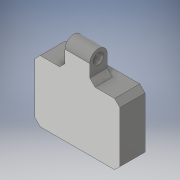
# Autodesk Inventor part: SDCardCover
Saved by Autodesk Inventor 2018 (Build 220112000, 112)
## iProperties
Created: 2019-01-13
Part Number: SDCardCover
Material: Generic
Document SubType Name: Modeling
Designer: tbrow
Density: 1 g/cm^3
Appearance: Default
Author: tbrow
## iProperties of the stored document SDCardCover_3DPrint.ipt
Created: 2019-01-15
Part Number: SDCardCover_3DPrint
Material: Generic
Document SubType Name: Modeling
Designer: tbrow
Density: 1 g/cm^3
Appearance: Default
Author: tbrow
Autodesk Inventor part; units mm, degrees
ref_plane "YZ Plane" through (0, 0, 0) normal (1, 0, 0) x (0, 1, 0)
ref_plane "XZ Plane" through (0, 0, 0) normal (0, 1, 0) x (-1, 0, 0)
ref_plane "XY Plane" through (0, 0, 0) normal (0, 0, 1) x (1, 0, 0)
sketch "Sketch1" plane through (0, 0, 0) normal (0, 0, 1) x (1, 0, 0)
  line L0 (0, 0) -> (0, 22.1234)
  line L1 (0, 22.1234) -> (10.795, 22.1234)
  line L2 (10.795, 22.1234) -> (10.795, 31.6484)
  line L3 (10.795, 31.6484) -> (19.685, 31.6484)
  line L4 (19.685, 31.6484) -> (19.685, 22.1234)
  line L5 (19.685, 22.1234) -> (30.48, 22.1234)
  line L6 (30.48, 22.1234) -> (30.48, 0)
  line L7 (30.48, 0) -> (0, 0)
  dimension "d0" = 10.795
  dimension "d1" = 9.525
  dimension "d2" = 8.89
  dimension "d3" = 10.795
  dimension "d17" = 31.6484
  constraints: 16 end point, 6 perpendicular, 2 point on line, 1 vertical
  measures "d0" distance of L4.end L5.end
  measures "d1" distance of L3.end L4.end
  measures "d2" distance of L2.end L3.end
  measures "d3" distance of L0.end L1.end
  measures "d17" distance between parallel lines of L7 L3
extrude "Extrusion1" add sketch "Sketch1" along normal blind 6.2484
sketch "Sketch2" plane through (19.685, 22.1234, 0) normal (1, 0, 0) x (0, 0, -1)
  circle A0 centre (-3.1242, 6.4008) radius 1.8542
  line L0 (0, 9.525) -> (-6.2484, 9.525) projected
  line L1 (-3.1242, 9.525) -> (-3.1242, 0) construction
  line L2 (0, 0) -> (-6.2484, 0) projected
  point P0 (0, -22.1234)
  dimension "d7" = 3.7084
  dimension "d8" = 3.1242
  constraints: 2 end point, 2 midpoint, 1 centre point, 1 point on line
  measures "d7" diameter of A0
  measures "d8" distance from line of L0 A0.centre
extrude "Extrusion2" cut sketch "Sketch2" against normal through all
fillet "Fillet1" radius 3.1242 2 edges at (15.24, 31.6484, 6.2484) (15.24, 31.6484, 0)
chamfer "Chamfer1" distance 1.905 angle 45 6 edges at (19.685, 22.1234, 3.1242) (10.795, 22.1234, 3.1242) (30.48, 22.1234, 3.1242) (0, 22.1234, 3.1242) (30.48, 0, 3.1242) (0, 0, 3.1242)
sketch "Sketch4" plane through (0, 0, 0) normal (0, 0, -1) x (-1, 0, 0)
  line L0 (-21.59, 22.1234) -> (-8.89, 22.1234)
  line L1 (-1.905, 22.1234) -> (-8.89, 22.1234) projected
  line L2 (-1.905, 22.1234) -> (0, 20.2184) projected
  line L3 (0, 1.905) -> (0, 20.2184) projected
  line L4 (0, 1.905) -> (-1.905, 0) projected
  line L5 (-28.575, 0) -> (-1.905, 0) projected
  line L6 (-28.575, 0) -> (-30.48, 1.905) projected
  line L7 (-30.48, 20.2184) -> (-30.48, 1.905) projected
  line L8 (-30.48, 20.2184) -> (-28.575, 22.1234) projected
  line L9 (-21.59, 22.1234) -> (-28.575, 22.1234) projected
  line L10 (-28.0489, 20.8534) -> (-29.21, 19.6923)
  line L11 (-29.21, 19.6923) -> (-29.21, 2.4311)
  line L12 (-29.21, 2.4311) -> (-28.0489, 1.27)
  line L13 (-28.0489, 1.27) -> (-2.4311, 1.27)
  line L14 (-2.4311, 1.27) -> (-1.27, 2.4311)
  line L15 (-1.27, 2.4311) -> (-1.27, 19.6923)
  line L16 (-1.27, 19.6923) -> (-2.4311, 20.8534)
  line L17 (-2.4311, 20.8534) -> (-8.89, 20.8534)
  line L18 (-8.89, 20.8534) -> (-21.59, 20.8534)
  line L19 (-21.59, 20.8534) -> (-28.0489, 20.8534)
  line L20 (-29.21, 3.175) -> (-1.27, 3.175)
  point P0 (0, 0)
  point P1 (-29.21, 3.81)
  point P2 (-30.48, 3.81)
  point P3 (-1.27, 3.81)
  point P4 (0, 3.81)
  dimension "d18" = 1.27
  dimension "d19" = 3.175
  constraints: 24 end point, 6 point on line, 1 horizontal, 1 perpendicular, 9 other
  measures "d18" distance between parallel lines of L9 L19
  measures "d19" distance between parallel lines of L20 L5
extrude "Extrusion3" add sketch "Sketch4" along normal blind 2.794
body "Solid1"
